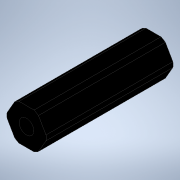
# Autodesk Inventor part: 9inthundershaft
Saved by Autodesk Inventor 2022 (Build 260153000, 153)
## iProperties
Created: 2020-01-14
Part Number: 9inthundershaft
Material: Aluminum 6061
Document SubType Name: Modeling
Designer: aidan
Density: 2.7 g/cm^3
Appearance: Anodized - Black
Author: aidan
Autodesk Inventor part; units mm, degrees
ref_plane "YZ Plane" through (0, 0, 0) normal (1, 0, 0) x (0, 1, 0)
ref_plane "XZ Plane" through (0, 0, 0) normal (0, 1, 0) x (-1, 0, 0)
ref_plane "XY Plane" through (0, 0, 0) normal (0, 0, 1) x (1, 0, 0)
sketch "Sketch1" plane through (0, 0, 0) normal (0, 0, 1) x (1, 0, 0)
  circle A0 centre (-2.6438, 6.9447) radius 6.8758
  line L0 (-9.4616, 7.8359) -> (-6.8245, 12.4034)
  line L1 (-6.8245, 1.4859) -> (-9.4616, 6.0534)
  line L2 (-0.0068, 0.5947) -> (-5.2808, 0.5947)
  line L3 (4.174, 6.0534) -> (1.537, 1.4859)
  line L4 (1.537, 12.4034) -> (4.174, 7.8359)
  line L5 (-5.2808, 13.2947) -> (-0.0068, 13.2947)
  point P0 (0, 0)
  point P1 (1.537, 1.4859)
  dimension "d0" = 13.7516
  dimension "d4" = 360
  constraints: 12 end point, 2 point on circle, 1 centre point, 1 coincident, 19 other
  measures "d0" diameter of A0
extrude "Extrusion1" add sketch "Sketch1" along normal blind 44.45 contours A0 L3 L2 L1 L0 L5 L4
sketch "Sketch2" plane through (0, 0, 44.45) normal (0, 0, 1) x (1, 0, 0)
  circle A0 centre (-2.6438, 6.9447) radius 2.5527
  line L0 (-5.2808, 0.5947) -> (-0.0068, 0.5947) projected
  line L1 (-2.6438, 6.9447) -> (-5.2808, 0.5947) construction
  line L2 (-2.6438, 6.9447) -> (-0.0068, 0.5947) construction
  point P0 (0, 0)
  dimension "d8" = 5.1054
  dimension "d9" = 6.35
  constraints: 4 end point, 1 centre point, 1 equal length
  measures "d8" diameter of A0
  measures "d9" distance from line of L0 L1.start
extrude "Extrusion2" cut sketch "Sketch2" against normal blind 44.45
equation "\"d6\" = d5"
equation "\"d10\" = d5"
equation "\"d5\" = 44.45"
body "Solid1"
